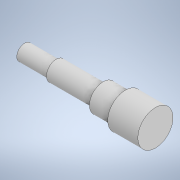
# Autodesk Inventor part: eixo com engenagem
Saved by Autodesk Inventor 2022.1 (Build 261234020, 234B)
## iProperties
Created: 2023-10-20
Part Number: eixo com engenagem
Material: Generic
Document SubType Name: Modeling
Designer: SENAI
Density: 1 g/cm^3
Appearance: Default
Author: SENAI
Autodesk Inventor part; units mm, degrees
ref_plane "YZ Plane" through (0, 0, 0) normal (1, 0, 0) x (0, 1, 0)
ref_plane "XZ Plane" through (0, 0, 0) normal (0, 1, 0) x (-1, 0, 0)
ref_plane "XY Plane" through (0, 0, 0) normal (0, 0, 1) x (1, 0, 0)
sketch "Sketch1" plane through (0, 0, 0) normal (0, 0, 1) x (1, 0, 0)
  line L0 (0, 0) -> (0, 10)
  line L1 (0, 10) -> (40.5, 10)
  line L2 (40.5, 12.5) -> (40.5, 10)
  line L3 (40.5, 12.5) -> (100.5, 12.5)
  line L4 (100.5, 17.5) -> (129, 17.5)
  line L5 (100.5, 17.5) -> (100.5, 12.5)
  line L6 (129, 17.5) -> (129, 22.5)
  line L7 (129, 22.5) -> (167.5, 22.5)
  line L8 (167.5, 22.5) -> (167.5, 0)
  line L9 (0, 0) -> (167.5, 0)
  dimension "d0" = 10
  dimension "d1" = 40.5
  dimension "d8" = 60
  dimension "d12" = 28.5
  dimension "d13" = 5
  dimension "d14" = 129
  dimension "d15" = 38.5
  constraints: 20 end point, 5 horizontal, 4 vertical, 1 perpendicular
  measures "d0" distance of L0.start L0.end
  measures "d1" distance of L0.end L1.end
  measures "d8" distance of L2.start L3.end
  measures "d12" distance of L4.start L4.end
  measures "d13" distance of L4.end L6.end
  measures "d14" horizontal distance of L6.end L0.end
  measures "d15" distance of L6.end L7.end
revolve "Revolution1" add sketch "Sketch1" angle 360 about axis through (0, 0, 0) along (1, 0, 0)
body "Solid1"
